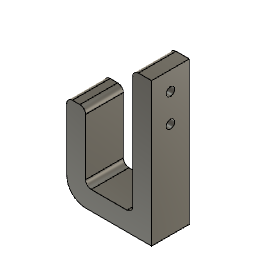
model-horizontal (Autodesk Fusion 360 design; units mm, degrees)
Autodesk Fusion 360 part; units mm, degrees
note: some values were not read from the file. Set by a fixed rule: which sketch regions a step uses.
sketch "Sketch1" plane through (0, 0, 0) normal (0, 1, 0) x (1, 0, 0)
  line L0 (10, -46) -> (10, -10)
  line L1 (10, -10) -> (35, -10)
  line L2 (35, -10) -> (35, -76)
  line L3 (35, -76) -> (45, -76)
  line L4 (45, -76) -> (45, 0)
  line L5 (45, 0) -> (0, 0)
  line L6 (0, 0) -> (0, -46)
  line L7 (0, -46) -> (10, -46)
  dimension "d1" = 36
  dimension "d2" = 25
  dimension "d3" = 10
  dimension "d4" = 10
  dimension "d5" = 10
  dimension "d6" = 30
  constraint vertical L0
  constraint perpendicular L0 L1
  constraint perpendicular L1 L2
  constraint perpendicular L2 L3
  constraint perpendicular L3 L4
  constraint coincident L5.end L6.start
  constraint perpendicular L2 L5
  constraint perpendicular L5 L6
  constraint perpendicular L6 L7
  measures "d1" distance of L0.start L0.end
  measures "d2" distance of L0.end L1.end
  measures "d3" distance of L2.end L3.end
  measures "d4" distance of L0.start L6.end
  measures "d5" distance of L1 L5
  measures "d6" distance of L3 L7
extrude "Extrude1" add sketch "Sketch1" along normal blind 20
sketch "Sketch2" plane through (35, 0, 0) normal (-1, 0, 0) x (0, -1, 0)
  line L0 (0, 10) -> (0, 76)
  line L1 (0, 76) -> (-20, 76)
  line L2 (-20, 76) -> (-20, 10)
  line L3 (-20, 10) -> (0, 10)
  circle A0 centre (-10, 66) radius 5
  circle A1 centre (-10, 51) radius 5
  line L4 (-20, 76) -> (-10, 66) construction
  line L5 (-10, 66) -> (0, 76) construction
  line L6 (-10, 66) -> (-10, 51) construction
  circle A2 centre (-10, 66) radius 2.25
  circle A3 centre (-10, 51) radius 2.25
  dimension "d9" = 10
  dimension "d11" = 15
  dimension "d12" = 10
  dimension "d13" = 10
  dimension "d14" = 4.5
  dimension "d15" = 4.5
  constraint coincident L1.end L2.start
  constraint coincident A0.centre L4.end
  constraint coincident L0.end L1.start
  constraint coincident A1.centre L6.end
  constraint vertical L6
  constraint equal L4 L5
  constraint concentric A0 A2
  constraint concentric A1 A3
  measures "d9" diameter of A0
  measures "d11" distance of A0.centre A1.centre
  measures "d12" vertical distance of A0.centre L1.end
  measures "d13" diameter of A1
  measures "d14" diameter of A2
  measures "d15" diameter of A3
extrude "Extrude2" cut sketch "Sketch2" against normal up to surface (10 mm away) contours A2 | A3
extrude "Extrude3" cut sketch "Sketch2" against normal blind 4 contours A0 | A1
chamfer "Chamfer1" distance 2.75 angle 45 2 edges at (39, 12.0977, 65.1864) (39, 12.0977, 50.1864)
fillet "Fillet2" radius 3 5 edges at (35, 10, 76) (35, 10, 10) (10, 10, 10) (10, 10, 46) (0, 10, 46)
fillet "Fillet2" radius 10 1 edges at (0, 10, 0)
equation "d13 = d9"
equation "d15 = d14"
